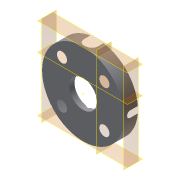
# Autodesk Inventor part: new end cap
Saved by Autodesk Inventor 2015 (Build 190159000, 159)
## iProperties
Created: 2014-09-13
Part Number: new end cap
Material: Generic
Document SubType Name: Modeling
Designer: jad211
Density: 1 g/cm^3
Appearance: Default
Author: jad211
Autodesk Inventor part; units mm, degrees
ref_plane "XZ Plane" through (0, 0, 0) normal (0, 1, 0) x (-1, 0, 0)
sketch "Sketch1" plane through (0, 0, 0) normal (0, 1, 0) x (-1, 0, 0)
  circle A0 centre (0, 0) radius 306.3875
  circle A1 centre (0, 0) radius 103.1875
  dimension "d0" = 612.775
  dimension "d1" = 206.375
  constraints: 2 centre point, 2 coincident
  measures "d0" diameter of A0
  measures "d1" diameter of A1
extrude "Extrusion1" add sketch "Sketch1" along normal blind 1
sketch "Sketch2" plane through (0, 1, 0) normal (0, 1, 0) x (1, 0, 0)
  circle A0 centre (0, 0) radius 306.3875
  circle A1 centre (0, 0) radius 305.8875
  dimension "d6" = 612.775
  dimension "d7" = 611.775
  constraints: 2 centre point, 1 coincident
  measures "d6" diameter of A0
  measures "d7" diameter of A1
extrude "Extrusion2" add sketch "Sketch2" along normal blind 101.6
sketch "Sketch3" plane through (0, 1, 0) normal (0, 1, 0) x (1, 0, 0)
  point P0 (0, 0)
sketch "Sketch4" plane through (0, 1, 0) normal (0, 1, 0) x (1, 0, 0)
  circle A0 centre (0, 0) radius 103.1875
  circle A1 centre (0, 0) radius 103.6875
  dimension "d10" = 206.375
  dimension "d11" = 207.375
  constraints: 2 centre point, 2 coincident
  measures "d10" diameter of A0
  measures "d11" diameter of A1
extrude "Extrusion3" add sketch "Sketch4" along normal blind 38.1
sketch "Sketch5" plane through (0, 1, 0) normal (0, 1, 0) x (1, 0, 0)
  circle A0 centre (-158.277, -158.277) radius 38.1
  circle A1 centre (-158.277, 158.277) radius 38.1
  circle A2 centre (158.277, 158.277) radius 38.1
  circle A3 centre (158.277, -158.4171) radius 38.1
  line L0 (-158.277, -158.277) -> (-158.277, 158.277) construction
  line L1 (-158.277, 158.277) -> (158.277, 158.277) construction
  line L2 (158.277, 158.277) -> (158.277, -158.277) construction
  line L3 (158.277, -158.277) -> (-158.277, -158.277) construction
  line L4 (-158.277, -158.277) -> (158.277, 158.277) construction
  line L5 (-158.277, 158.277) -> (158.277, -158.277) construction
  point P0 (0, 0)
  point P1 (0, 0)
  dimension "d15" = 76.2
  dimension "d16" = 76.2
  dimension "d17" = 76.2
  dimension "d18" = 76.2
  dimension "d19" = 316.554
  dimension "d20" = 316.554
  constraints: 12 end point, 4 centre point, 3 coincident, 3 midpoint, 2 parallel, 1 horizontal
  measures "d15" diameter of A0
  measures "d16" diameter of A1
  measures "d17" diameter of A2
  measures "d18" diameter of A3
  measures "d19" distance of L0.start L0.end
  measures "d20" distance of L0.end L1.end
extrude "Extrusion4" cut sketch "Sketch5" against normal blind 38.1
ref_plane "Work Plane1" through (-305.8875, 1, 0) normal (1, 0, 0) x (0, 1, 0)
sketch "Sketch6" plane through (-305.8875, 1, 0) normal (1, 0, 0) x (0, 1, 0)
  circle A0 centre (179.9908, 0) radius 111.9973
  point P0 (-1, 0)
  constraints: 1 centre point
extrude "Extrusion5" cut sketch "Sketch6" along normal mid plane 38.1
ref_plane "Work Plane2" through (305.8875, 1, 0) normal (1, 0, 0) x (0, 1, 0)
sketch "Sketch7" plane through (305.8875, 1, 0) normal (1, 0, 0) x (0, 1, 0)
  circle A0 centre (45.0104, 0) radius 24.1654
  point P0 (-1, 0)
  constraints: 1 centre point
extrude "Extrusion6" cut sketch "Sketch7" against normal blind 38.1 and the other way blind 19.05
ref_plane "Work Plane3" through (0, 0, 103.1875) normal (0, 0, 1) x (1, 0, 0)
sketch "Sketch8" plane through (0, 0, 103.1875) normal (0, 0, 1) x (1, 0, 0)
  circle A0 centre (0, 53.8641) radius 22.5449
  point P0 (0, 0)
  constraints: 1 centre point
extrude "Extrusion7" cut sketch "Sketch8" against normal blind 228.6 and the other way blind 1
sketch "Sketch9" plane through (0, 1, 0) normal (0, 1, 0) x (1, 0, 0)
  point P0 (0, 0)
ref_plane "Work Plane4" through (103.6875, 1, 0) normal (1, 0, 0) x (0, 1, 0)
sketch "Sketch10" plane through (103.6875, 1, 0) normal (1, 0, 0) x (0, 1, 0)
  circle A0 centre (50.5103, 0) radius 26.6834
  point P0 (-1, 0)
  constraints: 1 centre point
extrude "Extrusion8" cut sketch "Sketch10" against normal blind 76.2
ref_plane "Work Plane5" through (0, 0, 306.3875) normal (0, 0, 1) x (1, 0, 0)
sketch "Sketch11" plane through (0, 0, 306.3875) normal (0, 0, 1) x (1, 0, 0)
  circle A0 centre (0, 60) radius 50
  point P0 (0, 0)
  dimension "d35" = 100
  dimension "d36" = 60
  constraints: 1 centre point
  measures "d35" diameter of A0
  measures "d36" distance of point (0, 0) A0.centre
extrude "Extrusion9" cut sketch "Sketch11" against normal blind 76.2
sketch "Sketch12" plane through (0, 0, 306.3875) normal (0, 0, 1) x (1, 0, 0)
  line L0 (-50.3027, 145.9693) -> (50.3865, 146.5707)
  line L1 (50.3865, 146.5707) -> (50.3027, 59.2307)
  line L2 (50.3027, 59.2307) -> (-49.6973, 59.2307)
  line L3 (-49.6973, 59.2307) -> (-50.3027, 145.9693)
  line L4 (-295.7618, 102.6) -> (-295.7618, 102.6) projected
  line L5 (-50.3027, 145.9693) -> (50.3027, 59.2307) construction
  line L6 (50.3865, 146.5707) -> (-49.6973, 59.2307) construction
  point P0 (0, 0)
  point P1 (0, 102.6)
  point P2 (302.8958, 102.6)
  dimension "d39" = 100
  constraints: 12 end point, 1 midpoint, 1 point on line, 2 other
  measures "d39" distance of L1.end L2.end
extrude "Extrusion10" cut sketch "Sketch12" against normal blind 76.2
ref_plane "Work Plane6" through (0, 0, -306.3875) normal (0, 0, 1) x (1, 0, 0)
sketch "Sketch13" plane through (0, 0, -306.3875) normal (0, 0, 1) x (1, 0, 0)
  circle A0 centre (0, 60) radius 50
  point P0 (0, 0)
  dimension "d42" = 100
  dimension "d43" = 60
  constraints: 1 centre point
  measures "d42" diameter of A0
  measures "d43" distance of point (0, 0) A0.centre
extrude "Extrusion11" cut sketch "Sketch13" along normal blind 76.2
sketch "Sketch14" plane through (0, 0, -306.3875) normal (0, 0, 1) x (1, 0, 0)
  line L0 (-50, 116.7064) -> (50, 116.7064)
  line L1 (50, 116.7064) -> (50, 60)
  line L2 (50, 60) -> (-50, 60)
  line L3 (-50, 60) -> (-50, 116.7064)
  line L4 (-50, 116.7064) -> (50, 60) construction
  line L5 (50, 116.7064) -> (-50, 60) construction
  point P0 (0, 0)
  point P1 (0, 88.3532)
  dimension "d46" = 100
  dimension "d47" = 60
  constraints: 12 end point, 2 midpoint
  measures "d46" distance of L1.end L2.end
  measures "d47" distance from line of point (0, 0) L2
extrude "Extrusion12" cut sketch "Sketch14" along normal blind 76.2
sketch "Sketch15" plane through (305.8875, 1, 0) normal (1, 0, 0) x (0, 1, 0)
  line L0 (101.6, 301.7161) -> (101.6, -301.7734) projected
  line L1 (101.6, 23.6093) -> (42.299, 23.6093)
  line L2 (42.299, 23.6093) -> (42.299, -24.9083)
  line L3 (42.299, -24.9083) -> (101.6, -24.9083)
  line L4 (101.6, -24.9083) -> (101.6, 23.6093)
  point P0 (-1, 0)
  constraints: 8 end point, 1 point on line
extrude "Extrusion13" cut sketch "Sketch15" along normal blind 76.2 and the other way blind 38.1
equation "\"d16\" = d15"
equation "\"d17\" = d15"
equation "\"d18\" = d15"
equation "\"d20\" = d19"
body "Solid1"
